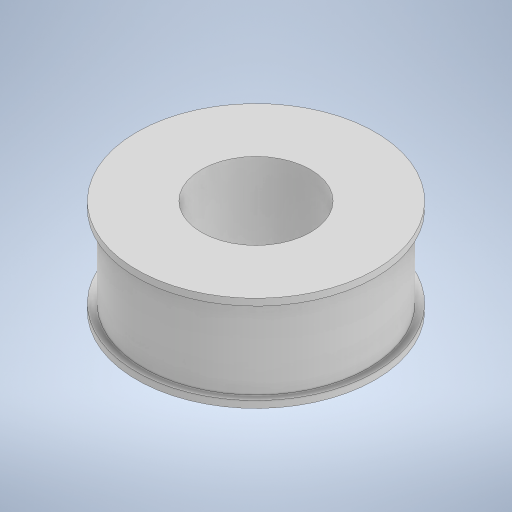
# Autodesk Inventor part: Подшипник
Saved by Autodesk Inventor 2023 (Build 270158000, 158)
## iProperties
Created: 2022-05-01
Part Number: Подшипник
Material: Типовые
Document SubType Name: Modeling
Designer: User
Density: 1 g/cm^3
Appearance: По умолчанию
Author: User
Autodesk Inventor part; units mm, degrees
ref_plane "YZ Plane" through (0, 0, 0) normal (1, 0, 0) x (0, 1, 0)
ref_plane "XZ Plane" through (0, 0, 0) normal (0, 1, 0) x (-1, 0, 0)
ref_plane "XY Plane" through (0, 0, 0) normal (0, 0, 1) x (1, 0, 0)
sketch "Эскиз1" plane through (0, 0, 0) normal (0, 1, 0) x (-1, 0, 0)
  circle A0 centre (0, 0) radius 8
  circle A1 centre (0, 0) radius 17.5
  dimension "d0" = 16
  dimension "d1" = 35
  constraints: 2 centre point, 2 coincident
  measures "d0" diameter of A0
  measures "d1" diameter of A1
extrude "Выдавливание1" add sketch "Эскиз1" along normal blind 14
sketch "Эскиз2" plane through (0, 0, 0) normal (0, 0, 1) x (1, 0, 0)
  line L0 (0, 0) -> (0, 14)
  line L1 (17.5, 14) -> (-17.5, 14) projected
  line L2 (0, 14) -> (17.5, 14)
  line L3 (17.5, 0) -> (17.5, 14) projected
  line L4 (17.5, 14) -> (17.5, 13)
  line L5 (17.5, 13) -> (16.5, 13)
  line L6 (17.5, 0) -> (0, 0)
  line L7 (17.5, 0) -> (-17.5, 0) projected
  line L8 (17.5, 0) -> (17.5, 1)
  line L9 (17.5, 1) -> (16.5, 1)
  line L10 (16.5, 1) -> (16.5, 13)
  dimension "d4" = 1
  dimension "d5" = 1
  dimension "d6" = 1
  dimension "d7" = 1
  constraints: 16 end point, 4 point on line, 3 perpendicular, 1 collinear, 1 midpoint
  measures "d4" distance of L2.end L4.end
  measures "d5" distance of L4.end L5.end
  measures "d6" distance of L6.start L8.end
  measures "d7" distance of L8.end L9.end
revolve "Вращение1" cut sketch "Эскиз2" angle 360 about axis through (0, 0, 0) along (0, 1, 0) keep common part contours L0 L1 L3 L5 L10 L9 L6
